Autodesk Fusion 360 part; units mm, degrees
(part 6 of 9)
sketch "Sketch11" plane through (0, 0, 0) normal (0, -1, 0) x (1, 0, 0)
  line L0 (123.2563, 74.675) -> (131.5375, 74.675)
  arc A0 (132.5375, 75.675) -> (131.5375, 74.675) centre (132.5375, 74.675) ccw
  line L1 (132.5375, 75.675) -> (138.5375, 75.675)
  arc A1 (139.5375, 74.675) -> (138.5375, 75.675) centre (138.5375, 74.675) ccw
  line L2 (139.5375, 74.675) -> (155.7375, 74.675)
  arc A2 (156.7375, 75.675) -> (155.7375, 74.675) centre (156.7375, 74.675) ccw
  line L3 (156.7375, 75.675) -> (162.7375, 75.675)
  arc A3 (163.7375, 74.675) -> (162.7375, 75.675) centre (162.7375, 74.675) ccw
  line L4 (163.7375, 74.675) -> (239.8875, 74.675)
  arc A4 (241.3625, 73.2) -> (239.8875, 74.675) centre (239.8875, 73.2) ccw
  line L5 (241.3625, 73.2) -> (241.3625, 58.15)
  arc A5 (241.3625, 58.15) -> (243.8875, 55.625) centre (243.8875, 58.15) ccw
  line L6 (243.8875, 55.625) -> (263.7, 55.625)
  arc A6 (265.175, 54.15) -> (263.7, 55.625) centre (263.7, 54.15) ccw
  line L7 (265.175, 54.15) -> (265.175, 3)
  arc A7 (263.7, 1.525) -> (265.175, 3) centre (263.7, 3) ccw
  line L8 (263.7, 1.525) -> (3, 1.525)
  arc A8 (1.525, 3) -> (3, 1.525) centre (3, 3) ccw
  line L9 (1.525, 3) -> (1.525, 54.15)
  arc A9 (3, 55.625) -> (1.525, 54.15) centre (3, 54.15) ccw
  line L10 (3, 55.625) -> (8.525, 55.625)
  arc A10 (8.525, 55.625) -> (11.05, 58.15) centre (8.525, 58.15) ccw
  line L11 (11.05, 58.15) -> (11.05, 73.2)
  arc A11 (12.525, 74.675) -> (11.05, 73.2) centre (12.525, 73.2) ccw
  line L12 (12.525, 74.675) -> (91.0563, 74.675)
  arc A12 (92.0563, 75.675) -> (91.0563, 74.675) centre (92.0563, 74.675) ccw
  line L13 (92.0563, 75.675) -> (98.0563, 75.675)
  arc A13 (99.0563, 74.675) -> (98.0563, 75.675) centre (98.0563, 74.675) ccw
  line L14 (99.0563, 74.675) -> (115.2563, 74.675)
  arc A14 (116.2563, 75.675) -> (115.2563, 74.675) centre (116.2563, 74.675) ccw
  line L15 (116.2563, 75.675) -> (122.2563, 75.675)
  arc A15 (123.2563, 74.675) -> (122.2563, 75.675) centre (122.2563, 74.675) ccw
  arc A16 (266.7, 54.15) -> (263.7, 57.15) centre (263.7, 54.15) ccw
  line L16 (263.7, 57.15) -> (243.8875, 57.15)
  arc A17 (242.8875, 58.15) -> (243.8875, 57.15) centre (243.8875, 58.15) ccw
  line L17 (242.8875, 58.15) -> (242.8875, 73.2)
  arc A18 (242.8875, 73.2) -> (239.8875, 76.2) centre (239.8875, 73.2) ccw
  line L18 (239.8875, 76.2) -> (12.525, 76.2)
  arc A19 (12.525, 76.2) -> (9.525, 73.2) centre (12.525, 73.2) ccw
  line L19 (9.525, 73.2) -> (9.525, 58.15)
  arc A20 (8.525, 57.15) -> (9.525, 58.15) centre (8.525, 58.15) ccw
  line L20 (8.525, 57.15) -> (3, 57.15)
  arc A21 (3, 57.15) -> (0, 54.15) centre (3, 54.15) ccw
  line L21 (0, 54.15) -> (0, 3)
  arc A22 (0, 3) -> (3, 0) centre (3, 3) ccw
  line L22 (3, 0) -> (263.7, 0)
  arc A23 (263.7, 0) -> (266.7, 3) centre (263.7, 3) ccw
  line L23 (266.7, 3) -> (266.7, 54.15)
  line L24 (5.3312, 47.625) -> (13.3312, 47.625)
  line L25 (13.3312, 47.625) -> (13.3312, 55.625)
  line L26 (12.3312, 56.625) -> (6.3312, 56.625)
  line L27 (5.3312, 55.625) -> (5.3312, 47.625)
  line L28 (5.3313, 53.625) -> (5.3312, 41.625)
  line L29 (37.5312, 50.468) -> (29.5312, 50.468)
  line L30 (29.5312, 50.468) -> (29.5312, 55.625)
  line L31 (30.5312, 56.625) -> (36.5312, 56.625)
  line L32 (37.5312, 55.625) -> (37.5312, 50.468)
  line L33 (37.5312, 41.625) -> (37.5312, 53.625)
  line L34 (36.5313, 54.625) -> (6.3312, 54.625)
  arc A24 (6.3312, 56.625) -> (5.3312, 55.625) centre (6.3312, 55.625) ccw
  arc A25 (13.3312, 55.625) -> (12.3312, 56.625) centre (12.3313, 55.625) ccw
  arc A26 (30.5312, 56.625) -> (29.5312, 55.625) centre (30.5312, 55.625) ccw
  arc A27 (37.5312, 55.625) -> (36.5313, 56.625) centre (36.5313, 55.625) ccw
  line L35 (22.6687, 35.575) -> (10.6688, 35.575)
  line L36 (23.6688, 22.575) -> (23.6687, 34.575)
  line L37 (38.5312, 40.625) -> (38.5312, 35.575)
  line L38 (4.3312, 35.575) -> (4.3312, 40.625)
  line L39 (48.8625, 35.575) -> (36.8625, 35.575)
  line L40 (5.3312, 43.3208) -> (5.3312, 40.625)
  line L41 (37.5312, 42.8695) -> (37.5312, 40.625)
  line L42 (9.6687, 33.1922) -> (7.8129, 33.1922)
  line L43 (7.8129, 33.1922) -> (7.8129, 35.575)
  line L44 (7.8129, 35.575) -> (8.6687, 35.575)
  line L45 (9.6688, 34.575) -> (9.6687, 33.1922)
  line L46 (9.6687, 34.575) -> (9.6687, 22.575)
  line L47 (23.6688, 32.8112) -> (25.1023, 32.8112)
  line L48 (25.1023, 32.8112) -> (25.1023, 35.575)
  line L49 (25.1023, 35.575) -> (24.6688, 35.575)
  line L50 (23.6687, 34.575) -> (23.6688, 32.8112)
  arc A28 (9.6688, 34.575) -> (8.6687, 35.575) centre (8.6687, 34.575) ccw
  arc A29 (24.6688, 35.575) -> (23.6687, 34.575) centre (24.6688, 34.575) ccw
  line L51 (38.5312, 35.575) -> (24.6687, 35.575)
  line L52 (19.1687, 35.575) -> (14.1687, 35.575)
  line L53 (8.6687, 35.575) -> (4.3312, 35.575)
  line L54 (4.3312, 40.625) -> (5.3312, 40.625)
  line L55 (37.5312, 40.625) -> (38.5312, 40.625)
  line L56 (18.9313, 54.625) -> (23.9313, 54.625)
  line L57 (23.9313, 54.625) -> (23.9313, 55.625)
  line L58 (23.9313, 55.625) -> (18.9313, 55.625)
  line L59 (18.9313, 55.625) -> (18.9313, 54.625)
  line L60 (9.6687, 33.1922) -> (23.6688, 32.8112)
  dimension "d166" = 8
  dimension "d167" = 8
  dimension "d168" = 2
  dimension "d169" = 2
  dimension "d170" = 1
  dimension "d171" = 5
  dimension "d173" = 4.5
  dimension "d174" = 1
  dimension "d175" = 1
  dimension "d176" = 1
  dimension "d177" = 1
  dimension "d178" = 5
  dimension "d179" = 1
  dimension "d180" = 13.6
  constraint horizontal L24
  constraint vertical L25
  constraint horizontal L26
  constraint vertical L27
  constraint midpoint L24.start L28
  constraint horizontal L29
  constraint vertical L30
  constraint horizontal L31
  constraint vertical L32
  constraint coincident L29.start L33
  constraint tangent L26 A24
  constraint tangent L27 A24
  constraint tangent L25 A25
  constraint tangent L26 A25
  constraint equal A24 A25
  constraint tangent L30 A26
  constraint tangent L31 A26
  constraint equal A24 A26
  constraint tangent L31 A27
  constraint tangent L32 A27
  constraint equal A24 A27
  constraint coincident L52.end L35
  constraint horizontal L54
  constraint vertical L37
  constraint horizontal L51
  constraint vertical L38
  constraint coincident L37.end L39
  constraint coincident L28 L40.start
  constraint perpendicular L40 L54
  constraint coincident L33 L41.start
  constraint perpendicular L41 L54
  constraint horizontal L42
  constraint vertical L43
  constraint horizontal L44
  constraint vertical L45
  constraint coincident L43.end L51
  constraint coincident L42.start L46
  constraint horizontal L47
  constraint vertical L48
  constraint horizontal L49
  constraint vertical L50
  constraint coincident L48.end L51
  constraint coincident L36 L47.start
  constraint tangent L44 A28
  constraint tangent L45 A28
  constraint tangent L49 A29
  constraint tangent L50 A29
  constraint collinear L51 L52
  constraint collinear L52 L53
  constraint collinear L54 L55
  constraint horizontal L56
  constraint vertical L57
  constraint horizontal L58
  constraint vertical L59
  constraint coincident L34 L56.start
  measures "d166" distance of L24.start L24.end
  measures "d167" distance of L29.start L29.end
  measures "d168" distance of L31 L34
  measures "d169" distance of L26 L34
  measures "d170" radius of A24
  measures "d171" distance of L52.end L52.start
  measures "d173" distance of L52.start L36
  measures "d174" distance of L33 L37
  measures "d175" distance of L28 L38
  measures "d176" radius of A28
  measures "d177" radius of A29
  measures "d178" distance of L56.start L56.end
  measures "d179" distance of L56.start L58.end
  measures "d180" distance of L33 L56.end
extrude "Extrude10" cut sketch "Sketch11" against normal blind 3.6 contours L10 A10 L24 L25 L26 L27 L28 A25 | L10 A10 L26 A24 | L24 L25 L28 L29 L30 L33 L34 L36 L37 L38 L39 L40 L41 L44 L45 L46 L49 L50 A28 A29 L51 L53 L54 L55 L56 L60 | L34 L56 L57 L58 L59 | L29 L30 L31 L32 L33 A26 A27
fillet "Fillet6" radius 1 2 edges at (4.3312, 2.1, 40.625) (38.5312, 2.1, 40.625)
fillet "Fillet7" radius 1 2 edges at (18.9313, 2.1, 55.625) (23.9313, 2.1, 55.625)
sketch "Sketch12" plane through (0, 0.6, 0) normal (0, -1, 0) x (1, 0, 0)
  arc A0 (65.4375, 54.625) -> (64.4375, 53.625) centre (65.4375, 53.625) ccw
  line L0 (65.4375, 54.625) -> (77.4375, 54.625)
  arc A1 (78.4375, 53.625) -> (77.4375, 54.625) centre (77.4375, 53.625) ccw
  line L1 (78.4375, 53.625) -> (78.4375, 41.625)
  arc A2 (77.4375, 40.625) -> (78.4375, 41.625) centre (77.4375, 41.625) ccw
  line L2 (77.4375, 40.625) -> (65.4375, 40.625)
  arc A3 (64.4375, 41.625) -> (65.4375, 40.625) centre (65.4375, 41.625) ccw
  line L3 (64.4375, 41.625) -> (64.4375, 53.625)
  arc A4 (198.7875, 73.675) -> (197.7875, 72.675) centre (198.7875, 72.675) ccw
  line L4 (198.7875, 73.675) -> (210.7875, 73.675)
  arc A5 (211.7875, 72.675) -> (210.7875, 73.675) centre (210.7875, 72.675) ccw
  line L5 (211.7875, 72.675) -> (211.7875, 60.675)
  arc A6 (210.7875, 59.675) -> (211.7875, 60.675) centre (210.7875, 60.675) ccw
  line L6 (210.7875, 59.675) -> (198.7875, 59.675)
  arc A7 (197.7875, 60.675) -> (198.7875, 59.675) centre (198.7875, 60.675) ccw
  line L7 (197.7875, 60.675) -> (197.7875, 72.675)
  arc A8 (244.0312, 54.625) -> (243.0313, 53.625) centre (244.0312, 53.625) ccw
  line L8 (244.0312, 54.625) -> (256.0312, 54.625)
  arc A9 (257.0312, 53.625) -> (256.0312, 54.625) centre (256.0312, 53.625) ccw
  line L9 (257.0312, 53.625) -> (257.0312, 41.625)
  arc A10 (256.0312, 40.625) -> (257.0312, 41.625) centre (256.0312, 41.625) ccw
  line L10 (256.0312, 40.625) -> (244.0312, 40.625)
  arc A11 (243.0313, 41.625) -> (244.0312, 40.625) centre (244.0312, 41.625) ccw
  line L11 (243.0312, 41.625) -> (243.0312, 53.625)
  arc A12 (14.4313, 60.675) -> (15.4313, 59.675) centre (15.4313, 60.675) ccw
  line L12 (14.4313, 60.675) -> (14.4313, 72.675)
  arc A13 (15.4313, 73.675) -> (14.4313, 72.675) centre (15.4313, 72.675) ccw
  line L13 (15.4313, 73.675) -> (27.4313, 73.675)
  arc A14 (28.4312, 72.675) -> (27.4313, 73.675) centre (27.4312, 72.675) ccw
  line L14 (28.4312, 72.675) -> (28.4313, 60.675)
  arc A15 (27.4313, 59.675) -> (28.4313, 60.675) centre (27.4313, 60.675) ccw
  line L15 (27.4313, 59.675) -> (15.4313, 59.675)
  arc A16 (165.45, 16.525) -> (164.45, 15.525) centre (165.45, 15.525) ccw
  line L16 (165.45, 16.525) -> (177.45, 16.525)
  arc A17 (178.45, 15.525) -> (177.45, 16.525) centre (177.45, 15.525) ccw
  line L17 (178.45, 15.525) -> (178.45, 3.525)
  arc A18 (177.45, 2.525) -> (178.45, 3.525) centre (177.45, 3.525) ccw
  line L18 (177.45, 2.525) -> (165.45, 2.525)
  arc A19 (164.45, 3.525) -> (165.45, 2.525) centre (165.45, 3.525) ccw
  line L19 (164.45, 3.525) -> (164.45, 15.525)
  arc A20 (67.8188, 73.675) -> (66.8188, 72.675) centre (67.8188, 72.675) ccw
  line L20 (67.8188, 73.675) -> (79.8188, 73.675)
  arc A21 (80.8188, 72.675) -> (79.8188, 73.675) centre (79.8188, 72.675) ccw
  line L21 (80.8187, 72.675) -> (80.8187, 60.675)
  arc A22 (79.8188, 59.675) -> (80.8188, 60.675) centre (79.8188, 60.675) ccw
  line L22 (79.8188, 59.675) -> (67.8188, 59.675)
  arc A23 (66.8188, 60.675) -> (67.8188, 59.675) centre (67.8188, 60.675) ccw
  line L23 (66.8188, 60.675) -> (66.8188, 72.675)
  arc A24 (261.3688, 34.575) -> (260.3688, 35.575) centre (260.3688, 34.575) ccw
  line L24 (261.3688, 34.575) -> (261.3688, 22.575)
  arc A25 (260.3688, 21.575) -> (261.3688, 22.575) centre (260.3688, 22.575) ccw
  line L25 (260.3688, 21.575) -> (230.1688, 21.575)
  arc A26 (229.1688, 22.575) -> (230.1688, 21.575) centre (230.1688, 22.575) ccw
  line L26 (229.1688, 22.575) -> (229.1688, 34.575)
  arc A27 (230.1688, 35.575) -> (229.1688, 34.575) centre (230.1688, 34.575) ccw
  line L27 (230.1688, 35.575) -> (260.3688, 35.575)
  arc A28 (184.5, 16.525) -> (183.5, 15.525) centre (184.5, 15.525) ccw
  line L28 (184.5, 16.525) -> (196.5, 16.525)
  arc A29 (197.5, 15.525) -> (196.5, 16.525) centre (196.5, 15.525) ccw
  line L29 (197.5, 15.525) -> (197.5, 3.525)
  arc A30 (196.5, 2.525) -> (197.5, 3.525) centre (196.5, 3.525) ccw
  line L30 (196.5, 2.525) -> (184.5, 2.525)
  arc A31 (183.5, 3.525) -> (184.5, 2.525) centre (184.5, 3.525) ccw
  line L31 (183.5, 3.525) -> (183.5, 15.525)
  arc A32 (45.1, 15.525) -> (44.1, 16.525) centre (44.1, 15.525) ccw
  line L32 (45.1, 15.525) -> (45.1, 3.525)
  arc A33 (44.1, 2.525) -> (45.1, 3.525) centre (44.1, 3.525) ccw
  line L33 (44.1, 2.525) -> (32.1, 2.525)
  arc A34 (31.1, 3.525) -> (32.1, 2.525) centre (32.1, 3.525) ccw
  line L34 (31.1, 3.525) -> (31.1, 15.525)
  arc A35 (32.1, 16.525) -> (31.1, 15.525) centre (32.1, 15.525) ccw
  line L35 (32.1, 16.525) -> (44.1, 16.525)
  arc A36 (55.9125, 35.575) -> (54.9125, 34.575) centre (55.9125, 34.575) ccw
  line L36 (55.9125, 35.575) -> (67.9125, 35.575)
  arc A37 (68.9125, 34.575) -> (67.9125, 35.575) centre (67.9125, 34.575) ccw
  line L37 (68.9125, 34.575) -> (68.9125, 22.575)
  arc A38 (67.9125, 21.575) -> (68.9125, 22.575) centre (67.9125, 22.575) ccw
  line L38 (67.9125, 21.575) -> (55.9125, 21.575)
  arc A39 (54.9125, 22.575) -> (55.9125, 21.575) centre (55.9125, 22.575) ccw
  line L39 (54.9125, 22.575) -> (54.9125, 34.575)
  arc A40 (46.3875, 54.625) -> (45.3875, 53.625) centre (46.3875, 53.625) ccw
  line L40 (46.3875, 54.625) -> (58.3875, 54.625)
  arc A41 (59.3875, 53.625) -> (58.3875, 54.625) centre (58.3875, 53.625) ccw
  line L41 (59.3875, 53.625) -> (59.3875, 41.625)
  arc A42 (58.3875, 40.625) -> (59.3875, 41.625) centre (58.3875, 41.625) ccw
  line L42 (58.3875, 40.625) -> (46.3875, 40.625)
  arc A43 (45.3875, 41.625) -> (46.3875, 40.625) centre (46.3875, 41.625) ccw
  line L43 (45.3875, 41.625) -> (45.3875, 53.625)
  arc A44 (70.2, 16.525) -> (69.2, 15.525) centre (70.2, 15.525) ccw
  line L44 (70.2, 16.525) -> (82.2, 16.525)
  arc A45 (83.2, 15.525) -> (82.2, 16.525) centre (82.2, 15.525) ccw
  line L45 (83.2, 15.525) -> (83.2, 3.525)
  arc A46 (82.2, 2.525) -> (83.2, 3.525) centre (82.2, 3.525) ccw
  line L46 (82.2, 2.525) -> (70.2, 2.525)
  arc A47 (69.2, 3.525) -> (70.2, 2.525) centre (70.2, 3.525) ccw
  line L47 (69.2, 3.525) -> (69.2, 15.525)
  arc A48 (172.5938, 73.675) -> (171.5938, 72.675) centre (172.5938, 72.675) ccw
  line L48 (172.5938, 73.675) -> (184.5938, 73.675)
  arc A49 (185.5937, 72.675) -> (184.5938, 73.675) centre (184.5937, 72.675) ccw
  line L49 (185.5937, 72.675) -> (185.5937, 60.675)
  arc A50 (184.5938, 59.675) -> (185.5937, 60.675) centre (184.5938, 60.675) ccw
  line L50 (184.5938, 59.675) -> (172.5937, 59.675)
  arc A51 (171.5938, 60.675) -> (172.5938, 59.675) centre (172.5938, 60.675) ccw
  line L51 (171.5937, 60.675) -> (171.5938, 72.675)
  arc A52 (151.1625, 35.575) -> (150.1625, 34.575) centre (151.1625, 34.575) ccw
  line L52 (151.1625, 35.575) -> (163.1625, 35.575)
  arc A53 (164.1625, 34.575) -> (163.1625, 35.575) centre (163.1625, 34.575) ccw
  line L53 (164.1625, 34.575) -> (164.1625, 22.575)
  arc A54 (163.1625, 21.575) -> (164.1625, 22.575) centre (163.1625, 22.575) ccw
  line L54 (163.1625, 21.575) -> (151.1625, 21.575)
  arc A55 (150.1625, 22.575) -> (151.1625, 21.575) centre (151.1625, 22.575) ccw
  line L55 (150.1625, 22.575) -> (150.1625, 34.575)
  arc A56 (89.25, 16.525) -> (88.25, 15.525) centre (89.25, 15.525) ccw
  line L56 (89.25, 16.525) -> (101.25, 16.525)
  arc A57 (102.25, 15.525) -> (101.25, 16.525) centre (101.25, 15.525) ccw
  line L57 (102.25, 15.525) -> (102.25, 3.525)
  arc A58 (101.25, 2.525) -> (102.25, 3.525) centre (101.25, 3.525) ccw
  line L58 (101.25, 2.525) -> (89.25, 2.525)
  arc A59 (88.25, 3.525) -> (89.25, 2.525) centre (89.25, 3.525) ccw
  line L59 (88.25, 3.525) -> (88.25, 15.525)
  arc A60 (41.625, 73.675) -> (40.625, 72.675) centre (41.625, 72.675) ccw
  line L60 (41.625, 73.675) -> (53.625, 73.675)
  arc A61 (54.625, 72.675) -> (53.625, 73.675) centre (53.625, 72.675) ccw
  line L61 (54.625, 72.675) -> (54.625, 60.675)
  arc A62 (53.625, 59.675) -> (54.625, 60.675) centre (53.625, 60.675) ccw
  line L62 (53.625, 59.675) -> (41.625, 59.675)
  arc A63 (40.625, 60.675) -> (41.625, 59.675) centre (41.625, 60.675) ccw
  line L63 (40.625, 60.675) -> (40.625, 72.675)
  arc A64 (74.9625, 35.575) -> (73.9625, 34.575) centre (74.9625, 34.575) ccw
  line L64 (74.9625, 35.575) -> (86.9625, 35.575)
  arc A65 (87.9625, 34.575) -> (86.9625, 35.575) centre (86.9625, 34.575) ccw
  line L65 (87.9625, 34.575) -> (87.9625, 22.575)
  arc A66 (86.9625, 21.575) -> (87.9625, 22.575) centre (86.9625, 22.575) ccw
  line L66 (86.9625, 21.575) -> (74.9625, 21.575)
  arc A67 (73.9625, 22.575) -> (74.9625, 21.575) centre (74.9625, 22.575) ccw
  line L67 (73.9625, 22.575) -> (73.9625, 34.575)
  arc A68 (227.3625, 16.525) -> (226.3625, 15.525) centre (227.3625, 15.525) ccw
  line L68 (227.3625, 16.525) -> (239.3625, 16.525)
  arc A69 (240.3625, 15.525) -> (239.3625, 16.525) centre (239.3625, 15.525) ccw
  line L69 (240.3625, 15.525) -> (240.3625, 3.525)
  arc A70 (239.3625, 2.525) -> (240.3625, 3.525) centre (239.3625, 3.525) ccw
  line L70 (239.3625, 2.525) -> (227.3625, 2.525)
  arc A71 (226.3625, 3.525) -> (227.3625, 2.525) centre (227.3625, 3.525) ccw
  line L71 (226.3625, 3.525) -> (226.3625, 15.525)
  arc A72 (208.3125, 35.575) -> (207.3125, 34.575) centre (208.3125, 34.575) ccw
  line L72 (208.3125, 35.575) -> (220.3125, 35.575)
  arc A73 (221.3125, 34.575) -> (220.3125, 35.575) centre (220.3125, 34.575) ccw
  line L73 (221.3125, 34.575) -> (221.3125, 22.575)
  arc A74 (220.3125, 21.575) -> (221.3125, 22.575) centre (220.3125, 22.575) ccw
  line L74 (220.3125, 21.575) -> (208.3125, 21.575)
  arc A75 (207.3125, 22.575) -> (208.3125, 21.575) centre (208.3125, 22.575) ccw
  line L75 (207.3125, 22.575) -> (207.3125, 34.575)
  arc A76 (8.2875, 16.525) -> (7.2875, 15.525) centre (8.2875, 15.525) ccw
  line L76 (8.2875, 16.525) -> (20.2875, 16.525)
  arc A77 (21.2875, 15.525) -> (20.2875, 16.525) centre (20.2875, 15.525) ccw
  line L77 (21.2875, 15.525) -> (21.2875, 3.525)
  arc A78 (20.2875, 2.525) -> (21.2875, 3.525) centre (20.2875, 3.525) ccw
  line L78 (20.2875, 2.525) -> (8.2875, 2.525)
  arc A79 (7.2875, 3.525) -> (8.2875, 2.525) centre (8.2875, 3.525) ccw
  line L79 (7.2875, 3.525) -> (7.2875, 15.525)
  arc A80 (51.15, 16.525) -> (50.15, 15.525) centre (51.15, 15.525) ccw
  line L80 (51.15, 16.525) -> (63.15, 16.525)
  arc A81 (64.15, 15.525) -> (63.15, 16.525) centre (63.15, 15.525) ccw
  line L81 (64.15, 15.525) -> (64.15, 3.525)
  arc A82 (63.15, 2.525) -> (64.15, 3.525) centre (63.15, 3.525) ccw
  line L82 (63.15, 2.525) -> (51.15, 2.525)
  arc A83 (50.15, 3.525) -> (51.15, 2.525) centre (51.15, 3.525) ccw
  line L83 (50.15, 3.525) -> (50.15, 15.525)
  arc A84 (198.7875, 54.625) -> (197.7875, 53.625) centre (198.7875, 53.625) ccw
  line L84 (198.7875, 54.625) -> (210.7875, 54.625)
  arc A85 (211.7875, 53.625) -> (210.7875, 54.625) centre (210.7875, 53.625) ccw
  line L85 (211.7875, 53.625) -> (211.7875, 41.625)
  arc A86 (210.7875, 40.625) -> (211.7875, 41.625) centre (210.7875, 41.625) ccw
  line L86 (210.7875, 40.625) -> (198.7875, 40.625)
  arc A87 (197.7875, 41.625) -> (198.7875, 40.625) centre (198.7875, 41.625) ccw
  line L87 (197.7875, 41.625) -> (197.7875, 53.625)
  arc A88 (224.9813, 73.675) -> (223.9813, 72.675) centre (224.9813, 72.675) ccw
  line L88 (224.9813, 73.675) -> (236.9813, 73.675)
  arc A89 (237.9812, 72.675) -> (236.9813, 73.675) centre (236.9813, 72.675) ccw
  line L89 (237.9812, 72.675) -> (237.9813, 60.675)
  arc A90 (236.9813, 59.675) -> (237.9813, 60.675) centre (236.9813, 60.675) ccw
  line L90 (236.9813, 59.675) -> (224.9813, 59.675)
  arc A91 (223.9812, 60.675) -> (224.9813, 59.675) centre (224.9813, 60.675) ccw
  line L91 (223.9812, 60.675) -> (223.9813, 72.675)
  arc A92 (170.2125, 35.575) -> (169.2125, 34.575) centre (170.2125, 34.575) ccw
  line L92 (170.2125, 35.575) -> (182.2125, 35.575)
  arc A93 (183.2125, 34.575) -> (182.2125, 35.575) centre (182.2125, 34.575) ccw
  line L93 (183.2125, 34.575) -> (183.2125, 22.575)
  arc A94 (182.2125, 21.575) -> (183.2125, 22.575) centre (182.2125, 22.575) ccw
  line L94 (182.2125, 21.575) -> (170.2125, 21.575)
  arc A95 (169.2125, 22.575) -> (170.2125, 21.575) centre (170.2125, 22.575) ccw
  line L95 (169.2125, 22.575) -> (169.2125, 34.575)
  arc A96 (127.35, 16.525) -> (126.35, 15.525) centre (127.35, 15.525) ccw
  line L96 (127.35, 16.525) -> (139.35, 16.525)
  arc A97 (140.35, 15.525) -> (139.35, 16.525) centre (139.35, 15.525) ccw
  line L97 (140.35, 15.525) -> (140.35, 3.525)
  arc A98 (139.35, 2.525) -> (140.35, 3.525) centre (139.35, 3.525) ccw
  line L98 (139.35, 2.525) -> (127.35, 2.525)
  arc A99 (126.35, 3.525) -> (127.35, 2.525) centre (127.35, 3.525) ccw
  line L99 (126.35, 3.525) -> (126.35, 15.525)
  arc A100 (113.0625, 35.575) -> (112.0625, 34.575) centre (113.0625, 34.575) ccw
  line L100 (113.0625, 35.575) -> (125.0625, 35.575)
  arc A101 (126.0625, 34.575) -> (125.0625, 35.575) centre (125.0625, 34.575) ccw
  line L101 (126.0625, 34.575) -> (126.0625, 22.575)
  arc A102 (125.0625, 21.575) -> (126.0625, 22.575) centre (125.0625, 22.575) ccw
  line L102 (125.0625, 21.575) -> (113.0625, 21.575)
  arc A103 (112.0625, 22.575) -> (113.0625, 21.575) centre (113.0625, 22.575) ccw
  line L103 (112.0625, 22.575) -> (112.0625, 34.575)
  arc A104 (146.4, 16.525) -> (145.4, 15.525) centre (146.4, 15.525) ccw
  line L104 (146.4, 16.525) -> (158.4, 16.525)
  arc A105 (159.4, 15.525) -> (158.4, 16.525) centre (158.4, 15.525) ccw
  line L105 (159.4, 15.525) -> (159.4, 3.525)
  arc A106 (158.4, 2.525) -> (159.4, 3.525) centre (158.4, 3.525) ccw
  line L106 (158.4, 2.525) -> (146.4, 2.525)
  arc A107 (145.4, 3.525) -> (146.4, 2.525) centre (146.4, 3.525) ccw
  line L107 (145.4, 3.525) -> (145.4, 15.525)
  arc A108 (189.2625, 35.575) -> (188.2625, 34.575) centre (189.2625, 34.575) ccw
  line L108 (189.2625, 35.575) -> (201.2625, 35.575)
  arc A109 (202.2625, 34.575) -> (201.2625, 35.575) centre (201.2625, 34.575) ccw
  line L109 (202.2625, 34.575) -> (202.2625, 22.575)
  arc A110 (201.2625, 21.575) -> (202.2625, 22.575) centre (201.2625, 22.575) ccw
  line L110 (201.2625, 21.575) -> (189.2625, 21.575)
  arc A111 (188.2625, 22.575) -> (189.2625, 21.575) centre (189.2625, 22.575) ccw
  line L111 (188.2625, 22.575) -> (188.2625, 34.575)
  arc A112 (203.55, 16.525) -> (202.55, 15.525) centre (203.55, 15.525) ccw
  line L112 (203.55, 16.525) -> (215.55, 16.525)
  arc A113 (216.55, 15.525) -> (215.55, 16.525) centre (215.55, 15.525) ccw
  line L113 (216.55, 15.525) -> (216.55, 3.525)
  arc A114 (215.55, 2.525) -> (216.55, 3.525) centre (215.55, 3.525) ccw
  line L114 (215.55, 2.525) -> (203.55, 2.525)
  arc A115 (202.55, 3.525) -> (203.55, 2.525) centre (203.55, 3.525) ccw
  line L115 (202.55, 3.525) -> (202.55, 15.525)
  arc A116 (108.3, 16.525) -> (107.3, 15.525) centre (108.3, 15.525) ccw
  line L116 (108.3, 16.525) -> (120.3, 16.525)
  arc A117 (121.3, 15.525) -> (120.3, 16.525) centre (120.3, 15.525) ccw
  line L117 (121.3, 15.525) -> (121.3, 3.525)
  arc A118 (120.3, 2.525) -> (121.3, 3.525) centre (120.3, 3.525) ccw
  line L118 (120.3, 2.525) -> (108.3, 2.525)
  arc A119 (107.3, 3.525) -> (108.3, 2.525) centre (108.3, 3.525) ccw
  line L119 (107.3, 3.525) -> (107.3, 15.525)
  arc A120 (179.7375, 54.625) -> (178.7375, 53.625) centre (179.7375, 53.625) ccw
  line L120 (179.7375, 54.625) -> (191.7375, 54.625)
  arc A121 (192.7375, 53.625) -> (191.7375, 54.625) centre (191.7375, 53.625) ccw
  line L121 (192.7375, 53.625) -> (192.7375, 41.625)
  arc A122 (191.7375, 40.625) -> (192.7375, 41.625) centre (191.7375, 41.625) ccw
  line L122 (191.7375, 40.625) -> (179.7375, 40.625)
  arc A123 (178.7375, 41.625) -> (179.7375, 40.625) centre (179.7375, 41.625) ccw
  line L123 (178.7375, 41.625) -> (178.7375, 53.625)
  arc A124 (217.8375, 54.625) -> (216.8375, 53.625) centre (217.8375, 53.625) ccw
  line L124 (217.8375, 54.625) -> (229.8375, 54.625)
  arc A125 (230.8375, 53.625) -> (229.8375, 54.625) centre (229.8375, 53.625) ccw
  line L125 (230.8375, 53.625) -> (230.8375, 41.625)
  arc A126 (229.8375, 40.625) -> (230.8375, 41.625) centre (229.8375, 41.625) ccw
  line L126 (229.8375, 40.625) -> (217.8375, 40.625)
  arc A127 (216.8375, 41.625) -> (217.8375, 40.625) centre (217.8375, 41.625) ccw
  line L127 (216.8375, 41.625) -> (216.8375, 53.625)
  arc A128 (251.175, 16.525) -> (250.175, 15.525) centre (251.175, 15.525) ccw
  line L128 (251.175, 16.525) -> (263.175, 16.525)
  arc A129 (264.175, 15.525) -> (263.175, 16.525) centre (263.175, 15.525) ccw
  line L129 (264.175, 15.525) -> (264.175, 3.525)
  arc A130 (263.175, 2.525) -> (264.175, 3.525) centre (263.175, 3.525) ccw
  line L130 (263.175, 2.525) -> (251.175, 2.525)
  arc A131 (250.175, 3.525) -> (251.175, 2.525) centre (251.175, 3.525) ccw
  line L131 (250.175, 3.525) -> (250.175, 15.525)
  arc A132 (132.1125, 35.575) -> (131.1125, 34.575) centre (132.1125, 34.575) ccw
  line L132 (132.1125, 35.575) -> (144.1125, 35.575)
  arc A133 (145.1125, 34.575) -> (144.1125, 35.575) centre (144.1125, 34.575) ccw
  line L133 (145.1125, 34.575) -> (145.1125, 22.575)
  arc A134 (144.1125, 21.575) -> (145.1125, 22.575) centre (144.1125, 22.575) ccw
  line L134 (144.1125, 21.575) -> (132.1125, 21.575)
  arc A135 (131.1125, 22.575) -> (132.1125, 21.575) centre (132.1125, 22.575) ccw
  line L135 (131.1125, 22.575) -> (131.1125, 34.575)
  arc A136 (94.0125, 35.575) -> (93.0125, 34.575) centre (94.0125, 34.575) ccw
  line L136 (94.0125, 35.575) -> (106.0125, 35.575)
  arc A137 (107.0125, 34.575) -> (106.0125, 35.575) centre (106.0125, 34.575) ccw
  line L137 (107.0125, 34.575) -> (107.0125, 22.575)
  arc A138 (106.0125, 21.575) -> (107.0125, 22.575) centre (106.0125, 22.575) ccw
  line L138 (106.0125, 21.575) -> (94.0125, 21.575)
  arc A139 (93.0125, 22.575) -> (94.0125, 21.575) centre (94.0125, 22.575) ccw
  line L139 (93.0125, 22.575) -> (93.0125, 34.575)
  circle A140 centre (128.588, 37.025) radius 2
  circle A141 centre (220.025, 66.675) radius 2
  circle A142 centre (47.625, 9.525) radius 2
  circle A143 centre (245.269, 9.525) radius 2
  circle A144 centre (32.525, 66.675) radius 2
  line L140 (36.8625, 35.575) -> (24.6688, 35.575)
  arc A145 (24.6688, 35.575) -> (23.6687, 34.575) centre (24.6688, 34.575) ccw
  line L141 (23.6687, 34.575) -> (23.6688, 22.575)
  arc A146 (22.6687, 21.575) -> (23.6688, 22.575) centre (22.6688, 22.575) ccw
  line L142 (22.6687, 21.575) -> (10.6688, 21.575)
  arc A147 (9.6687, 22.575) -> (10.6688, 21.575) centre (10.6687, 22.575) ccw
  line L143 (9.6687, 22.575) -> (9.6687, 34.575)
  arc A148 (9.6687, 34.575) -> (8.6687, 35.575) centre (8.6687, 34.575) ccw
  line L144 (8.6687, 35.575) -> (4.3312, 35.575)
  line L145 (4.3312, 35.575) -> (4.3313, 39.625)
  arc A149 (5.3312, 40.625) -> (4.3312, 39.625) centre (5.3312, 39.625) ccw
  line L146 (5.3312, 40.625) -> (5.3312, 55.625)
  line L147 (5.3312, 55.625) -> (3, 55.625)
  arc A150 (3, 55.625) -> (1.525, 54.15) centre (3, 54.15) ccw
  line L148 (1.525, 54.15) -> (1.525, 3)
  arc A151 (1.525, 3) -> (3, 1.525) centre (3, 3) ccw
  line L149 (3, 1.525) -> (263.7, 1.525)
  arc A152 (263.7, 1.525) -> (265.175, 3) centre (263.7, 3) ccw
  line L150 (265.175, 3) -> (265.175, 54.15)
  arc A153 (265.175, 54.15) -> (263.7, 55.625) centre (263.7, 54.15) ccw
  line L151 (263.7, 55.625) -> (243.8875, 55.625)
  arc A154 (241.3625, 58.15) -> (243.8875, 55.625) centre (243.8875, 58.15) ccw
  line L152 (241.3625, 58.15) -> (241.3625, 73.2)
  arc A155 (241.3625, 73.2) -> (239.8875, 74.675) centre (239.8875, 73.2) ccw
  line L153 (239.8875, 74.675) -> (163.7375, 74.675)
  line L154 (163.7375, 74.675) -> (163.7375, 59.675)
  arc A156 (164.7375, 58.675) -> (163.7375, 59.675) centre (163.7375, 58.675) ccw
  line L155 (164.7375, 58.675) -> (164.7375, 55.625)
  line L156 (164.7375, 55.625) -> (168.1875, 55.625)
  arc A157 (169.1875, 54.625) -> (168.1875, 55.625) centre (168.1875, 54.625) ccw
  line L157 (169.1875, 54.625) -> (172.6875, 54.625)
  arc A158 (173.6875, 53.625) -> (172.6875, 54.625) centre (172.6875, 53.625) ccw
  line L158 (173.6875, 53.625) -> (173.6875, 41.625)
  arc A159 (172.6875, 40.625) -> (173.6875, 41.625) centre (172.6875, 41.625) ccw
  line L159 (172.6875, 40.625) -> (160.6875, 40.625)
  arc A160 (159.6875, 41.625) -> (160.6875, 40.625) centre (160.6875, 41.625) ccw
  line L160 (159.6875, 41.625) -> (159.6875, 53.625)
  arc A161 (159.6875, 53.625) -> (158.6875, 54.625) centre (158.6875, 53.625) ccw
  line L161 (158.6875, 54.625) -> (155.6375, 54.625)
  arc A162 (155.6375, 54.625) -> (154.6375, 53.625) centre (155.6375, 53.625) ccw
  line L162 (154.6375, 53.625) -> (154.6375, 41.625)
  arc A163 (153.6375, 40.625) -> (154.6375, 41.625) centre (153.6375, 41.625) ccw
  line L163 (153.6375, 40.625) -> (141.6375, 40.625)
  arc A164 (140.6375, 41.625) -> (141.6375, 40.625) centre (141.6375, 41.625) ccw
  line L164 (140.6375, 41.625) -> (140.6375, 53.625)
  arc A165 (140.6375, 53.625) -> (139.6375, 54.625) centre (139.6375, 53.625) ccw
  line L165 (139.6375, 54.625) -> (136.5875, 54.625)
  arc A166 (136.5875, 54.625) -> (135.5875, 53.625) centre (136.5875, 53.625) ccw
  line L166 (135.5875, 53.625) -> (135.5875, 41.625)
  arc A167 (134.5875, 40.625) -> (135.5875, 41.625) centre (134.5875, 41.625) ccw
  line L167 (134.5875, 40.625) -> (122.5875, 40.625)
  arc A168 (121.5875, 41.625) -> (122.5875, 40.625) centre (122.5875, 41.625) ccw
  line L168 (121.5875, 41.625) -> (121.5875, 53.625)
  arc A169 (121.5875, 53.625) -> (120.5875, 54.625) centre (120.5875, 53.625) ccw
  line L169 (120.5875, 54.625) -> (117.5375, 54.625)
  arc A170 (117.5375, 54.625) -> (116.5375, 53.625) centre (117.5375, 53.625) ccw
  line L170 (116.5375, 53.625) -> (116.5375, 41.625)
  arc A171 (115.5375, 40.625) -> (116.5375, 41.625) centre (115.5375, 41.625) ccw
  line L171 (115.5375, 40.625) -> (103.5375, 40.625)
  arc A172 (102.5375, 41.625) -> (103.5375, 40.625) centre (103.5375, 41.625) ccw
  line L172 (102.5375, 41.625) -> (102.5375, 53.625)
  arc A173 (102.5375, 53.625) -> (101.5375, 54.625) centre (101.5375, 53.625) ccw
  line L173 (101.5375, 54.625) -> (98.4875, 54.625)
  arc A174 (98.4875, 54.625) -> (97.4875, 53.625) centre (98.4875, 53.625) ccw
  line L174 (97.4875, 53.625) -> (97.4875, 41.625)
  arc A175 (96.4875, 40.625) -> (97.4875, 41.625) centre (96.4875, 41.625) ccw
  line L175 (96.4875, 40.625) -> (84.4875, 40.625)
  arc A176 (83.4875, 41.625) -> (84.4875, 40.625) centre (84.4875, 41.625) ccw
  line L176 (83.4875, 41.625) -> (83.4875, 53.625)
  arc A177 (84.4875, 54.625) -> (83.4875, 53.625) centre (84.4875, 53.625) ccw
  line L177 (84.4875, 54.625) -> (87.9875, 54.625)
  arc A178 (88.9875, 55.625) -> (87.9875, 54.625) centre (88.9875, 54.625) ccw
  line L178 (88.9875, 55.625) -> (90.0563, 55.625)
  line L179 (90.0563, 55.625) -> (90.0563, 58.675)
  arc A179 (91.0563, 59.675) -> (90.0563, 58.675) centre (91.0563, 58.675) ccw
  line L180 (91.0563, 59.675) -> (91.0563, 74.675)
  line L181 (91.0563, 74.675) -> (12.525, 74.675)
  arc A180 (12.525, 74.675) -> (11.05, 73.2) centre (12.525, 73.2) ccw
  line L182 (11.05, 73.2) -> (11.05, 58.15)
  arc A181 (10.5375, 56.625) -> (11.05, 58.15) centre (8.525, 58.15) ccw
  line L183 (10.5375, 56.625) -> (12.3312, 56.625)
  arc A182 (13.3312, 55.625) -> (12.3312, 56.625) centre (12.3312, 55.625) ccw
  line L184 (13.3312, 55.625) -> (13.3312, 54.625)
  line L185 (13.3312, 54.625) -> (18.9313, 54.625)
  arc A183 (19.9313, 55.625) -> (18.9313, 54.625) centre (19.9313, 54.625) ccw
  line L186 (19.9313, 55.625) -> (22.9313, 55.625)
  arc A184 (23.9313, 54.625) -> (22.9313, 55.625) centre (22.9313, 54.625) ccw
  line L187 (23.9313, 54.625) -> (29.5312, 54.625)
  line L188 (29.5312, 54.625) -> (29.5312, 55.625)
  arc A185 (30.5312, 56.625) -> (29.5312, 55.625) centre (30.5312, 55.625) ccw
  line L189 (30.5312, 56.625) -> (36.5312, 56.625)
  arc A186 (37.5312, 55.625) -> (36.5312, 56.625) centre (36.5312, 55.625) ccw
  line L190 (37.5312, 55.625) -> (37.5312, 40.625)
  arc A187 (38.5312, 39.625) -> (37.5312, 40.625) centre (37.5312, 39.625) ccw
  line L191 (38.5312, 39.625) -> (38.5312, 35.575)
  line L192 (38.5312, 35.575) -> (48.8625, 35.575)
  arc A188 (49.8625, 34.575) -> (48.8625, 35.575) centre (48.8625, 34.575) ccw
  line L193 (49.8625, 34.575) -> (49.8625, 22.575)
  arc A189 (48.8625, 21.575) -> (49.8625, 22.575) centre (48.8625, 22.575) ccw
  line L194 (48.8625, 21.575) -> (36.8625, 21.575)
  arc A190 (35.8625, 22.575) -> (36.8625, 21.575) centre (36.8625, 22.575) ccw
  line L195 (35.8625, 22.575) -> (35.8625, 34.575)
  arc A191 (36.8625, 35.575) -> (35.8625, 34.575) centre (36.8625, 34.575) ccw
  line L196 (45.3625, 35.575) -> (38.3625, 35.575)
  line L197 (38.3625, 35.575) -> (38.3625, 36.575)
  line L198 (38.3625, 36.575) -> (45.3625, 36.575)
  line L199 (45.3625, 36.575) -> (45.3625, 35.575)
  line L200 (35.8625, 33.3924) -> (33.7425, 33.3924)
  line L201 (33.7425, 33.3924) -> (33.7425, 35.575)
  line L202 (33.7425, 35.575) -> (34.8625, 35.575)
  line L203 (35.8625, 34.575) -> (35.8625, 33.3924)
  arc A192 (35.8625, 34.575) -> (34.8625, 35.575) centre (34.8625, 34.575) ccw
  dimension "d185" = 7
  dimension "d186" = 1
  dimension "d187" = 4.5
  dimension "d188" = 1
  constraint horizontal L196
  constraint vertical L197
  constraint horizontal L198
  constraint vertical L199
  constraint coincident L192 L196.start
  constraint horizontal L200
  constraint vertical L201
  constraint horizontal L202
  constraint vertical L203
  constraint coincident L140 L201.end
  constraint coincident L195 L200.start
  constraint tangent L202 A192
  constraint tangent L203 A192
  measures "d185" distance of L196.start L196.end
  measures "d186" distance of L196.start L198.end
  measures "d187" distance of L193 L196.start
  measures "d188" radius of A192
extrude "Extrude11" cut sketch "Sketch12" against normal blind 3 contours L140 A191 A192 | L191 L192 L196 L198 L199
fillet "Fillet8" radius 1 1 edges at (45.3625, 2.1, 36.575)